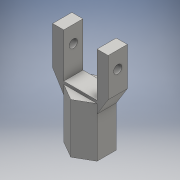
# Autodesk Inventor part: supportrodv1.2
Saved by Autodesk Inventor 2016 (Build 200138000, 138)
## iProperties
Created: 2016-05-22
Part Number: supportrodv1.2
Material: Generic
Document SubType Name: Modeling
Designer: Thetheos
Density: 1 g/cm^3
Appearance: Default
Author: Thetheos
Autodesk Inventor part; units mm, degrees
ref_plane "YZ Plane" through (0, 0, 0) normal (1, 0, 0) x (0, 1, 0)
ref_plane "XZ Plane" through (0, 0, 0) normal (0, 1, 0) x (-1, 0, 0)
ref_plane "XY Plane" through (0, 0, 0) normal (0, 0, 1) x (1, 0, 0)
sketch "Sketch1" plane through (0, 0, 0) normal (0, 0, 1) x (1, 0, 0)
  line L0 (8, 0.0718) -> (2, 3.5359)
  line L1 (2, 3.5359) -> (2, 10.4641)
  line L2 (2, 10.4641) -> (8, 13.9282)
  line L3 (8, 13.9282) -> (14, 10.4641)
  line L4 (14, 10.4641) -> (14, 3.5359)
  line L5 (14, 3.5359) -> (8, 0.0718)
  point P0 (0, 0)
  point P1 (8, 7)
  dimension "d1" = 12
  constraints: 12 end point, 13 other
  measures "d1" distance between parallel lines of L4 L1
extrude "Extrusion1" add sketch "Sketch1" along normal blind 18
sketch "Sketch2" plane through (0, 0, 0) normal (0, 0, -1) x (-1, 0, 0)
  circle A0 centre (-8, 7) radius 3.1
  point P0 (0, 0)
  dimension "d5" = 6.2
  constraints: 1 centre point
  measures "d5" diameter of A0
extrude "Extrusion2" cut sketch "Sketch2" against normal blind 14
sketch "Sketch3" plane through (0, 0, 18) normal (0, 0, 1) x (1, 0, 0)
  line L0 (14, 3.5359) -> (8, 0.0718) projected
  line L1 (14, 3.5359) -> (2, 3.5359)
  line L2 (2, 3.5359) -> (2, 10.4641)
  line L3 (2, 10.4641) -> (14, 10.4641)
  line L4 (14, 10.4641) -> (14, 3.5359)
  point P0 (0, 0)
  dimension "d12" = 6.9282
  constraints: 8 end point, 3 perpendicular, 1 horizontal
  measures "d12" distance between parallel lines of L3 L1
extrude "Extrusion3" add sketch "Sketch3" along normal blind 17
sketch "Sketch4" plane through (2, 10.4641, 18) normal (0, 1, 0) x (1, 0, 0)
  line L0 (12, 0) -> (12, -17) projected
  line L1 (12, -17) -> (16, -17)
  line L2 (0, 0) -> (0, -17) projected
  line L3 (12, 0) -> (12, -17)
  line L4 (0, -17) -> (-4, -17)
  line L5 (0, 0) -> (0, -17)
  line L6 (16, -17) -> (16, -3.1957)
  line L7 (-4, -3.1957) -> (0, 3.2792)
  line L8 (16, -3.1957) -> (12, 3.2792)
  line L9 (12, 18) -> (12, 0) projected
  line L10 (0, 0) -> (0, 3.2792)
  line L11 (12, 0) -> (12, 3)
  line L12 (-4, -17) -> (-4, -3.1957)
  point P0 (-2, 18)
  dimension "d10" = 4
  dimension "d11" = 4
  constraints: 20 end point, 3 collinear, 3 point on line, 2 vertical, 1 perpendicular
  measures "d10" distance of L0.end L1.end
  measures "d11" distance of L2.end L4.end
extrude "Extrusion4" add sketch "Sketch4" against normal blind 6.9282
sketch "Sketch5" plane through (2, 10.4641, 18) normal (0, 1, 0) x (1, 0, 0)
  line L0 (16, -17) -> (16, -17) projected
  line L1 (0, -17) -> (12, -17)
  line L2 (12, -17) -> (12, -1)
  line L3 (12, -1) -> (0, -1)
  line L4 (0, -1) -> (0, -17)
  point P0 (-2, 18)
  point P1 (-4, -17)
  constraints: 8 end point, 2 parallel, 1 horizontal, 1 perpendicular, 2 other
extrude "Extrusion5" cut sketch "Sketch5" against normal through all
sketch "Sketch6" plane through (-2, 10.4641, 21.1957) normal (-1, 0, 0) x (0, 0, 1)
  line L0 (13.8043, 0) -> (13.8043, -6.9282) projected
  circle A0 centre (7.8043, -3.4641) radius 1.5
  point P0 (-21.1957, -10.4641)
  dimension "d18" = 3
  constraints: 1 centre point
  measures "d18" diameter of A0
extrude "Extrusion6" cut sketch "Sketch6" against normal through all
body "Solid1"
